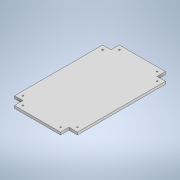
# Autodesk Inventor part: top
Saved by Autodesk Inventor 2020 (Build 240168000, 168)
## iProperties
Created: 2019-11-30
Part Number: top
Material: Générique
Document SubType Name: Modeling
Designer: bapti
Density: 1 g/cm^3
Appearance: Par défaut
Author: bapti
Autodesk Inventor part; units mm, degrees
ref_plane "YZ Plane" through (0, 0, 0) normal (1, 0, 0) x (0, 1, 0)
ref_plane "XZ Plane" through (0, 0, 0) normal (0, 1, 0) x (-1, 0, 0)
ref_plane "XY Plane" through (0, 0, 0) normal (0, 0, 1) x (1, 0, 0)
sketch "Esquisse1" plane through (0, 0, 0) normal (0, 1, 0) x (-1, 0, 0)
  line L0 (0, 0) -> (150, 0)
  line L1 (150, 0) -> (150, -250)
  line L2 (150, -250) -> (0, -250)
  line L3 (0, -250) -> (0, 0)
  line L4 (20, 0) -> (20, -20)
  line L5 (20, -20) -> (0, -20)
  line L6 (150, 0) -> (0, -250) construction
  line L7 (150, -250) -> (0, 0) construction
  line L8 (75, 0) -> (75, -250) construction
  line L9 (150, -125) -> (0, -125) construction
  line L10 (130, 0) -> (130, -20)
  line L11 (130, -20) -> (150, -20)
  line L12 (20, -250) -> (20, -230)
  line L13 (20, -230) -> (0, -230)
  line L14 (130, -250) -> (130, -230)
  line L15 (130, -230) -> (150, -230)
  circle A0 centre (30, -10) radius 1.65
  line L16 (20, -20) -> (0, 0) construction
  line L17 (0, -20) -> (20, 0) construction
  line L18 (30, -10) -> (20, -10) construction
  circle A1 centre (10, -30) radius 1.65
  circle A2 centre (120, -10) radius 1.65
  circle A3 centre (140, -30) radius 1.65
  circle A4 centre (30, -240) radius 1.65
  circle A5 centre (10, -220) radius 1.65
  circle A6 centre (120, -240) radius 1.65
  circle A7 centre (140, -220) radius 1.65
  dimension "d0" = 150
  dimension "d1" = 250
  dimension "d5" = 20
  dimension "d6" = 3.3
  dimension "d7" = 10
  dimension "d9" = 10
  constraints: 38 end point, 16 symmetric about line, 8 centre point, 5 midpoint, 5 perpendicular, 2 parallel, 2 point on line, 1 horizontal, 1 vertical, 7 other
  measures "d0" distance of L1.end L2.end
  measures "d1" distance of L2.end L0.start
  measures "d5" distance of L4.end L5.end
  measures "d6" diameter of A0
  measures "d7" distance of L18.start L18.end
  measures "d9" distance of L4.end L18.end
extrude "Extrusion1" add sketch "Esquisse1" along normal blind 6 contours L0 L10 L11 L1 L15 L14 L2 L12 L13 L3 L5 L4
